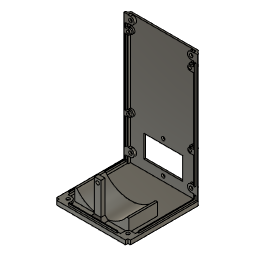
SolderingStation_Back (Autodesk Fusion 360 design; units mm, degrees)
Autodesk Fusion 360 part; units mm, degrees
sketch "Sketch1" plane through (0, 0, 0) normal (0, 0, 1) x (1, 0, 0)
  line L0 (45, 45) -> (-45, 45)
  line L1 (-45, 45) -> (-45, -45)
  line L2 (-45, -45) -> (45, -45)
  line L3 (45, -45) -> (45, 45)
  line L4 (45, 45) -> (-45, -45) construction
  line L5 (-45, 45) -> (45, -45) construction
  line L6 (-45, 45) -> (-42, 45) construction
  line L7 (-42, 45) -> (-42, 42)
  line L8 (-42, 42) -> (-45, 42)
  line L9 (0, 45) -> (0, -45) construction
  line L10 (-45, 0) -> (45, 0) construction
  line L11 (42, 45) -> (42, 42)
  line L12 (42, 42) -> (45, 42)
  line L13 (42, -42) -> (45, -42)
  line L14 (42, -45) -> (42, -42)
  line L15 (-42, -45) -> (-42, -42)
  line L16 (-42, -42) -> (-45, -42)
  dimension "d1" = 90
  dimension "d2" = 90
  constraint horizontal L0
  constraint perpendicular L0 L1
  constraint parallel L0 L2
  constraint parallel L1 L3
  constraint coincident L4 origin
  constraint coincident L5 origin
  constraint coincident L0 L6.end
  constraint coincident L5 L7.end
  constraint perpendicular L0 L7
  constraint coincident L1 L8.end
  constraint perpendicular L1 L8
  constraint midpoint L0 L9.start
  constraint midpoint L2 L9.end
  constraint midpoint L1 L10.start
  constraint midpoint L3 L10.end
  constraint symmetric L6.end L9 L11.start
  constraint symmetric L7.end L9 L11.end
  constraint symmetric L8.end L9 L12.end
  constraint symmetric L6.end L10 L15.start
  constraint symmetric L7.end L10 L15.end
  constraint symmetric L8.end L10 L16.end
  constraint symmetric L10 L11.start L14.start
  constraint symmetric L10 L11.end L13.start
  constraint symmetric L10 L12.end L13.end
  measures "d1" distance of L1.end L2.end
  measures "d2" distance of L0.end L1.end
extrude "Extrude1" add sketch "Sketch1" along normal blind 5 contours L0 L1 L2 L3 L7 L8 L11 L12 L13 L14 L15 L16 makes body 1
sketch "Sketch2" plane through (0, 0, 5) normal (0, 0, 1) x (-1, 0, 0)
  line L0 (42, 45) -> (-42, 45)
  line L1 (-42, 45) -> (-42, 42)
  line L2 (-42, 42) -> (-45, 42)
  line L3 (-45, 42) -> (-45, -42)
  line L4 (-45, -42) -> (-42, -42)
  line L5 (-42, -42) -> (-42, -45)
  line L6 (-42, -45) -> (42, -45)
  line L7 (42, -45) -> (42, -42)
  line L8 (42, -42) -> (45, -42)
  line L9 (45, -42) -> (45, 42)
  line L10 (45, 42) -> (42, 42)
  line L11 (42, 42) -> (42, 45)
  line L12 (38, -38) -> (41, -38)
  line L13 (41, -38) -> (41, 38)
  line L14 (41, 38) -> (38, 38)
  line L15 (38, 38) -> (38, 41)
  line L16 (38, 41) -> (-38, 41)
  line L17 (-38, 41) -> (-38, 38)
  line L18 (-38, 38) -> (-41, 38)
  line L19 (-41, 38) -> (-41, -38)
  line L20 (-41, -38) -> (-38, -38)
  line L21 (-38, -38) -> (-38, -41)
  line L22 (-38, -41) -> (38, -41)
  line L23 (38, -41) -> (38, -38)
  dimension "d5" = -4
extrude "Extrude2" cut sketch "Sketch2" against normal blind 3 contours L12 L13 L14 L15 L16 L17 L18 L19 L20 L21 L22 L23 bodies 1
sketch "Sketch3" plane through (0, 0, 5) normal (0, 0, 1) x (-1, 0, 0)
  line L0 (42, 45) -> (-42, 45)
  line L1 (-42, 45) -> (-42, 42)
  line L2 (-42, 42) -> (-45, 42)
  line L3 (-45, 42) -> (-45, -42)
  line L4 (-45, -42) -> (-42, -42)
  line L5 (-42, -42) -> (-42, -45)
  line L6 (-42, -45) -> (42, -45)
  line L7 (42, -45) -> (42, -42)
  line L8 (42, -42) -> (45, -42)
  line L9 (45, -42) -> (45, 42)
  line L10 (45, 42) -> (42, 42)
  line L11 (42, 42) -> (42, 45)
  line L12 (-39, 39) -> (-39, 42)
  line L13 (-39, 42) -> (39, 42)
  line L14 (39, 42) -> (39, 39)
  line L15 (39, 39) -> (42, 39)
  line L16 (42, 39) -> (42, -39)
  line L17 (42, -39) -> (39, -39)
  line L18 (39, -39) -> (39, -42)
  line L19 (39, -42) -> (-39, -42)
  line L20 (-39, -42) -> (-39, -39)
  line L21 (-39, -39) -> (-42, -39)
  line L22 (-42, -39) -> (-42, 39)
  line L23 (-42, 39) -> (-39, 39)
  line L24 (-40, 40) -> (-40, 43)
  line L25 (-40, 43) -> (40, 43)
  line L26 (40, 43) -> (40, 40)
  line L27 (40, 40) -> (43, 40)
  line L28 (43, 40) -> (43, -40)
  line L29 (43, -40) -> (40, -40)
  line L30 (40, -40) -> (40, -43)
  line L31 (40, -43) -> (-40, -43)
  line L32 (-40, -43) -> (-40, -40)
  line L33 (-40, -40) -> (-43, -40)
  line L34 (-43, -40) -> (-43, 40)
  line L35 (-43, 40) -> (-40, 40)
  line L36 (42, -39) -> (42, -40)
  line L37 (-42, -39) -> (-42, -40)
  line L38 (41, -38) -> (38, -38)
  line L39 (38, -38) -> (38, -41)
  line L40 (38, -41) -> (-38, -41)
  line L41 (-38, -41) -> (-38, -38)
  line L42 (-38, -38) -> (-41, -38)
  line L43 (-41, -38) -> (-41, 38)
  line L44 (-41, 38) -> (-38, 38)
  line L45 (-38, 38) -> (-38, 41)
  line L46 (-38, 41) -> (38, 41)
  line L47 (38, 41) -> (38, 38)
  line L48 (38, 38) -> (41, 38)
  line L49 (41, 38) -> (41, -38)
  constraint coincident L29 L36.end
  constraint perpendicular L29 L36
  constraint coincident L33 L37.end
  constraint perpendicular L33 L37
extrude "Extrude3" add sketch "Sketch3" along normal blind 2 contours L12 L13 L14 L15 L16 L22 L23 L24 L25 L26 L27 L28 L29 L33 L34 L35 L36 L37 bodies 1
fillet "Fillet1" radius 1 7 edges at (-42, 0.5, 5) (42, 0.5, 5) (40.5, -39, 5) (39, -40.5, 5) (0, -42, 5) (-39, -40.5, 5) (-40.5, -39, 5) on bodies 1
sketch "Sketch4" plane through (0, 0, 0) normal (0, 0, -1) x (1, 0, 0)
  line L0 (42, 45) -> (-42, 45)
  line L1 (-42, 45) -> (-42, 42)
  line L2 (-42, 42) -> (-45, 42)
  line L3 (-45, 42) -> (-45, -42)
  line L4 (-45, -42) -> (-42, -42)
  line L5 (-42, -42) -> (-42, -45)
  line L6 (-42, -45) -> (42, -45)
  line L7 (42, -45) -> (42, -42)
  line L8 (42, -42) -> (45, -42)
  line L9 (45, -42) -> (45, 42)
  line L10 (45, 42) -> (42, 42)
  line L11 (42, 42) -> (42, 45)
  line L12 (-45, -40) -> (-40, -40)
  line L13 (-40, -40) -> (-40, -43)
  line L14 (-40, -43) -> (40, -43)
  line L15 (40, -43) -> (40, -40)
  line L16 (40, -40) -> (45, -40)
  dimension "d14" = -2
extrude "Extrude4" add sketch "Sketch4" against normal blind 160 contours L3 L4 L5 L6 L7 L8 L9 L12 L13 L14 L15 L16 bodies 1
extrude "Extrude5" cut 1 faces at (-12.6667, 42.3333, 5) along direction (0, 0, -1) blind 3 on bodies 1 bodies 1
sketch "Sketch5" plane through (0, 0, 2) normal (0, 0, 1) x (-1, 0, 0)
  line L0 (41, -40) -> (41, 38)
  line L1 (41, 38) -> (38, 38)
  line L2 (38, 38) -> (38, 41)
  line L3 (38, 41) -> (-38, 41)
  line L4 (-38, 41) -> (-38, 38)
  line L5 (-38, 38) -> (-41, 38)
  line L6 (-41, 38) -> (-41, -40)
  line L7 (-41, -40) -> (-40, -40)
  line L8 (-40, -40) -> (-40, -43)
  line L9 (-40, -43) -> (40, -43)
  line L10 (40, -43) -> (40, -40)
  line L11 (40, -40) -> (41, -40)
  line L12 (-44.9376, -44.9376) -> (44.9376, -44.9376) construction
  line L13 (44.9376, -44.9376) -> (44.9376, 44.9376) construction
  line L14 (44.9376, 44.9376) -> (-44.9376, 44.9376) construction
  line L15 (-44.9376, 44.9376) -> (-44.9376, -44.9376) construction
  line L16 (-44.9376, -44.9376) -> (44.9376, 44.9376) construction
  line L17 (44.9376, -44.9376) -> (-44.9376, 44.9376) construction
  circle A0 centre (36.4523, 36.4523) radius 2.15 construction
  circle A1 centre (36.4523, 36.4523) radius 2.15 construction
  circle A2 centre (36.4523, 36.4523) radius 2
  line L18 (0, 0) -> (0, 44.9376) construction
  circle A3 centre (-36.4523, 36.4523) radius 2.15 construction
  circle A4 centre (-36.4523, 36.4523) radius 2
  dimension "d19" = 4.3
  dimension "d20" = 12
  dimension "d27" = 4.3
  constraint horizontal L12
  constraint perpendicular L12 L13
  constraint parallel L12 L14
  constraint parallel L13 L15
  constraint coincident L16 L18.start
  constraint coincident L17 L18.start
  constraint coincident L18.start origin
  constraint coincident L16 A0.centre
  constraint concentric A0 A1
  constraint concentric A0 A2
  constraint midpoint L14 L18.end
  constraint symmetric A1 L18 A3
  constraint concentric A3 A4
  measures "d19" diameter of A0
  measures "d20" distance of L13.end A0.centre
  measures "d27" diameter of A3
extrude "Extrude6" cut sketch "Sketch5" against normal blind 3 contours A2 | A4 bodies 1
sketch "Sketch7" plane through (0, 0, 0) normal (0, 0, -1) x (1, 0, 0)
  circle A0 centre (-36.4523, 36.4523) radius 2
  circle A1 centre (36.4523, 36.4523) radius 2
  line L0 (45, -42) -> (45, 42)
  line L1 (45, 42) -> (42, 42)
  line L2 (42, 42) -> (42, 45)
  line L3 (42, 45) -> (-42, 45)
  line L4 (-42, 45) -> (-42, 42)
  line L5 (-42, 42) -> (-45, 42)
  line L6 (-45, 42) -> (-45, -42)
  line L7 (-45, -42) -> (-42, -42)
  line L8 (-42, -42) -> (-42, -45)
  line L9 (-42, -45) -> (42, -45)
  line L10 (42, -45) -> (42, -42)
  line L11 (42, -42) -> (45, -42)
  circle A2 centre (-36.4523, 36.4523) radius 4.5
  line L12 (-36.4523, 36.4523) -> (-31.9523, 36.4523) construction
  line L13 (-36.4523, 36.4523) -> (-36.4523, 31.9523) construction
  line L14 (-31.9523, 36.4523) -> (-31.9523, 45)
  line L15 (-36.4523, 31.9523) -> (-45, 31.9523)
  line L16 (43, -42) -> (43, 40)
  line L17 (43, 40) -> (40, 40)
  line L18 (40, 40) -> (40, 43)
  line L19 (40, 43) -> (-40, 43)
  line L20 (-40, 43) -> (-40, 40)
  line L21 (-40, 40) -> (-43, 40)
  line L22 (-43, 40) -> (-43, -42)
  line L23 (0, 45) -> (0, 26) construction
  circle A3 centre (36.4523, 36.4523) radius 4.5
  line L24 (31.9523, 36.4523) -> (31.9523, 45)
  line L25 (36.4523, 31.9523) -> (45, 31.9523)
  dimension "d23" = 9
  dimension "d24" = -2
  constraint concentric A0 A2
  constraint coincident A0.centre A2.centre
  constraint coincident A2 L12.end
  constraint horizontal L12
  constraint coincident A2 L13.end
  constraint perpendicular L12 L13
  constraint coincident L3 L14.end
  constraint tangent A2 L14
  constraint coincident L6 L15.end
  constraint tangent A2 L15
  constraint midpoint L3 L23.start
  constraint perpendicular L3 L23
  constraint symmetric A2 L23 A3
  constraint symmetric L12.end L23 L24.start
  constraint symmetric L13.end L23 L25.start
  constraint symmetric L14.end L23 L24.end
  constraint symmetric L15.end L23 L25.end
  measures "d23" diameter of A2
extrude "Extrude7" add sketch "Sketch7" against normal blind 7 contours L16 L17 L18 L19 A3 L24 L25 | A3 | A2 L14 L15 L19 L20 L21 L22 | A2 bodies 1
sketch "Sketch9" plane through (0, 45, 0) normal (0, 1, 0) x (-1, 0, 0)
  line L0 (-42, 0) -> (42, 0)
  line L1 (42, 0) -> (42, 160)
  line L2 (42, 160) -> (-42, 160)
  line L3 (-42, 160) -> (-42, 0)
  line L4 (0, 0) -> (0, 67.5) construction
  line L5 (23.65, 41.15) -> (-23.65, 41.15)
  line L6 (-23.65, 41.15) -> (-23.65, 13.85)
  line L7 (-23.65, 13.85) -> (23.65, 13.85)
  line L8 (23.65, 13.85) -> (23.65, 41.15)
  line L9 (23.65, 41.15) -> (-23.65, 13.85) construction
  line L10 (-23.65, 41.15) -> (23.65, 13.85) construction
  circle A0 centre (0, 47.2) radius 2.15
  line L11 (0, 27.5) -> (-23.65, 27.5) construction
  circle A1 centre (0, 7.8) radius 2.15
  point P0 (0, 27.5)
  dimension "d28" = 47.3
  dimension "d29" = 27.3
  dimension "d30" = 27.5
  dimension "d31" = 4.3
  dimension "d33" = 19.7
  constraint coincident L4.start origin
  constraint perpendicular L0 L4
  constraint horizontal L5
  constraint perpendicular L5 L6
  constraint parallel L5 L7
  constraint parallel L6 L8
  constraint coincident L9 P0
  constraint coincident L10 P0
  constraint coincident L4 P0
  constraint coincident L4 A0.centre
  constraint coincident P0 L11.start
  constraint midpoint L6 L11.end
  constraint symmetric A0 L11 A1
  measures "d28" distance of L6.end L7.end
  measures "d29" distance of L5.end L6.end
  measures "d30" distance of L0 P0
  measures "d31" diameter of A0
  measures "d33" distance of A0.centre L11
extrude "Extrude8" cut sketch "Sketch9" against normal blind 2 contours L5 L6 L7 L8 | A0 | A1 bodies 1
sketch "Sketch10" plane through (0, 45, 0) normal (0, 1, 0) x (-1, 0, 0)
  circle A0 centre (0, 7.8) radius 2.15
  line L0 (-23.65, 41.15) -> (23.65, 41.15)
  line L1 (23.65, 41.15) -> (23.65, 13.85)
  line L2 (23.65, 13.85) -> (-23.65, 13.85)
  line L3 (-23.65, 13.85) -> (-23.65, 41.15)
  circle A1 centre (0, 47.2) radius 2.15
  line L4 (-42, 0) -> (42, 0)
  line L5 (42, 0) -> (42, 160)
  line L6 (42, 160) -> (-42, 160)
  line L7 (-42, 160) -> (-42, 0)
  circle A2 centre (-37, 15) radius 4.5
  line L8 (-45, 0) -> (-45, 160)
  circle A3 centre (-37, 15) radius 2.15
  line L9 (-37, 15) -> (-37, 19.5) construction
  line L10 (-37, 15) -> (-37, 10.5) construction
  line L11 (-37, 19.5) -> (-42, 19.5)
  line L12 (-37, 10.5) -> (-42, 10.5)
  line L13 (0, 0) -> (0, 47.2) construction
  circle A4 centre (37, 15) radius 4.5
  circle A5 centre (37, 15) radius 2.15
  line L14 (37, 10.5) -> (42, 10.5)
  line L15 (37, 19.5) -> (42, 19.5)
  circle A6 centre (37, 15) radius 2.15
  circle A7 centre (37, 15) radius 4.5
  line L16 (37, 19.5) -> (42, 19.5)
  line L17 (37, 10.5) -> (42, 10.5)
  line L18 (-37, 19.5) -> (-42, 19.5)
  circle A8 centre (-37, 15) radius 4.5
  circle A9 centre (-37, 15) radius 2.15
  circle A10 centre (-37, 155) radius 4.5
  line L19 (-37, 150.5) -> (-42, 150.5)
  circle A11 centre (-37, 155) radius 2.15
  line L20 (-37, 159.5) -> (-42, 159.5)
  line L21 (37, 150.5) -> (42, 150.5)
  circle A12 centre (37, 155) radius 4.5
  line L22 (37, 159.5) -> (42, 159.5)
  circle A13 centre (37, 155) radius 2.15
  dimension "d36" = 9
  dimension "d37" = 15
  dimension "d38" = 8
  dimension "d39" = 4.3
  dimension "d40" = 9
  dimension "d41" = 4.3
  dimension "d42" = 9
  dimension "d43" = 4.3
  constraint concentric A2 A3
  constraint coincident A2.centre A3.centre
  constraint coincident A2 L9.end
  constraint vertical L9
  constraint coincident A2 L10.end
  constraint parallel L9 L10
  constraint coincident L7 L11.end
  constraint tangent A2 L11
  constraint coincident L7 L12.end
  constraint tangent A2 L12
  constraint coincident L13.start origin
  constraint coincident A1.centre L13.end
  constraint symmetric A2 L13 A4
  constraint symmetric A3 L13 A5
  constraint symmetric L9.end L13 L15.start
  constraint symmetric L10.end L13 L14.start
  constraint symmetric L11.end L13 L15.end
  constraint symmetric L12.end L13 L14.end
  constraint concentric A8 A9
  constraint coincident L9.end A8
  constraint tangent L18 A8
  constraint concentric A10 A11
  constraint coincident L20.start A10
  constraint tangent A10 L20
  measures "d36" diameter of A2
  measures "d37" distance of L4 A2.centre
  measures "d38" distance of A2.centre L8
  measures "d39" diameter of A3
  measures "d40" diameter of A8
  measures "d41" diameter of A9
  measures "d42" diameter of A10
  measures "d43" diameter of A11
extrude "Extrude9" add sketch "Sketch10" against normal blind 7 contours L7 A2 L11 L12 L18 A8 | L5 A4 L14 L15 A7 L16 L17 | A2 A8 | A4 A7 | L7 A10 L19 L20 | L5 L21 A12 L22 | A10 | A12 bodies 1
sketch "Sketch11" plane through (0, 40, 0) normal (0, -1, 0) x (1, 0, 0)
  line L0 (40, 19.5) -> (42, 19.5)
  line L1 (42, 19.5) -> (42, 10.5)
  line L2 (42, 10.5) -> (40, 10.5)
  line L3 (40, 10.5) -> (40, 2)
  line L4 (40, 2) -> (41, 2)
  line L5 (41, 2) -> (41, 5)
  arc A0 (41, 5) -> (42, 6) centre (41, 6) ccw
  line L6 (42, 6) -> (42, 7)
  line L7 (42, 7) -> (43, 7)
  line L8 (43, 7) -> (43, 5)
  line L9 (43, 5) -> (45, 5)
  line L10 (45, 5) -> (45, 160)
  line L11 (45, 160) -> (40, 160)
  line L12 (40, 160) -> (40, 159.5)
  line L13 (40, 159.5) -> (42, 159.5)
  line L14 (42, 159.5) -> (42, 150.5)
  line L15 (42, 150.5) -> (40, 150.5)
  line L16 (40, 150.5) -> (40, 19.5)
  line L17 (43, 5) -> (43, 160)
  line L18 (42, 5) -> (42, 160)
  line L19 (0, 41) -> (0, 14) construction
  line L20 (-42, 5) -> (-42, 160)
  line L21 (-43, 5) -> (-43, 160)
  line L22 (-42, 5) -> (-43, 5)
  line L23 (-43, 160) -> (-42, 160)
  constraint coincident L8.end L9.start
  constraint coincident L11 L17.end
  constraint perpendicular L11 L17
  constraint coincident L11 L18.end
  constraint perpendicular L11 L18
  constraint vertical L19
  constraint vertical L20
  constraint parallel L20 L21
  constraint perpendicular L21 L22
  constraint perpendicular L20 L23
extrude "Extrude10" add sketch "Sketch11" along normal blind 2 contours L1 L7 L11 L14 L17 L18 | L20 L21 L22 L23 bodies 1
fillet "Fillet2" radius 1 6 edges at (-41.7071, 40, 5.2929) (-42, 40, 8.25) (-42, 40, 85) (42, 40, 85) (41.7071, 40, 5.2929) (42, 40, 8.25) on bodies 1
extrude "Extrude11" cut 4 faces at (37.6599, 43, 15.5763) (-36.4428, 43, 14.7238) (-36.6417, 43, 155.6207) (36.4461, 43, 155.5603) along direction (0, 1, 0) blind 2 on bodies 1 bodies 1
sketch "Sketch12" plane through (0, 0, 0) normal (0, 0, -1) x (1, 0, 0)
  circle A0 centre (-36.4523, 36.4523) radius 2
  circle A1 centre (36.4523, 36.4523) radius 2
  line L0 (45, -42) -> (45, 42)
  line L1 (45, 42) -> (42, 42)
  line L2 (42, 42) -> (42, 45)
  line L3 (42, 45) -> (-42, 45)
  line L4 (-42, 45) -> (-42, 42)
  line L5 (-42, 42) -> (-45, 42)
  line L6 (-45, 42) -> (-45, -42)
  line L7 (-45, -42) -> (-42, -42)
  line L8 (-42, -42) -> (-42, -45)
  line L9 (-42, -45) -> (42, -45)
  line L10 (42, -45) -> (42, -42)
  line L11 (42, -42) -> (45, -42)
  circle A2 centre (-36.4523, 36.4523) radius 3.75
  circle A3 centre (36.4523, 36.4523) radius 3.75
  dimension "d52" = 7.5
  dimension "d53" = 7.5
  constraint concentric A0 A2
  constraint concentric A1 A3
  measures "d52" diameter of A2
  measures "d53" diameter of A3
extrude "Extrude12" cut sketch "Sketch12" against normal blind 3 contours A2 | A3 bodies 1
sketch "Sketch13" plane through (0, 45, 0) normal (0, 1, 0) x (-1, 0, 0)
  circle A0 centre (37, 155) radius 2.15
  circle A1 centre (-37, 15) radius 2.15
  circle A2 centre (37, 15) radius 2.15
  circle A3 centre (-37, 155) radius 2.15
  circle A4 centre (0, 47.2) radius 2.15
  line L0 (-23.65, 41.15) -> (23.65, 41.15)
  line L1 (23.65, 41.15) -> (23.65, 13.85)
  line L2 (23.65, 13.85) -> (-23.65, 13.85)
  line L3 (-23.65, 13.85) -> (-23.65, 41.15)
  circle A5 centre (0, 7.8) radius 2.15
  line L4 (-42, 160) -> (-42, 0)
  line L5 (-42, 0) -> (42, 0)
  line L6 (42, 0) -> (42, 160)
  line L7 (42, 160) -> (-42, 160)
  circle A6 centre (-37, 155) radius 3.75
  circle A7 centre (37, 155) radius 3.75
  circle A8 centre (37, 15) radius 3.75
  circle A9 centre (-37, 15) radius 3.75
  dimension "d56" = 7.5
  dimension "d57" = 7.5
  dimension "d58" = 7.5
  dimension "d59" = 7.5
  constraint concentric A3 A6
  constraint concentric A0 A7
  constraint concentric A2 A8
  constraint concentric A1 A9
  measures "d56" diameter of A6
  measures "d57" diameter of A7
  measures "d58" diameter of A8
  measures "d59" diameter of A9
extrude "Extrude13" cut sketch "Sketch13" against normal blind 3 contours A6 | A7 | A8 | A9 bodies 1
sketch "Sketch14" plane through (0, 43, 0) normal (0, -1, 0) x (1, 0, 0)
  line L0 (37, 19.5) -> (40, 19.5)
  line L1 (40, 19.5) -> (40, 150.5)
  line L2 (40, 150.5) -> (37, 150.5)
  arc A0 (37, 159.5) -> (37, 150.5) centre (37, 155) ccw
  line L3 (37, 159.5) -> (40, 159.5)
  line L4 (40, 159.5) -> (40, 160)
  line L5 (40, 160) -> (-40, 160)
  line L6 (-40, 160) -> (-40, 159.5)
  line L7 (-40, 159.5) -> (-37, 159.5)
  arc A1 (-37, 150.5) -> (-37, 159.5) centre (-37, 155) ccw
  line L8 (-37, 150.5) -> (-40, 150.5)
  line L9 (-40, 150.5) -> (-40, 19.5)
  line L10 (-40, 19.5) -> (-37, 19.5)
  arc A2 (-37, 10.5) -> (-37, 19.5) centre (-37, 15) ccw
  line L11 (-37, 10.5) -> (-40, 10.5)
  line L12 (-40, 10.5) -> (-40, 2)
  line L13 (-40, 2) -> (40, 2)
  line L14 (40, 2) -> (40, 10.5)
  line L15 (40, 10.5) -> (37, 10.5)
  arc A3 (37, 19.5) -> (37, 10.5) centre (37, 15) ccw
  circle A4 centre (0, 47.2) radius 2.15
  line L16 (-23.65, 41.15) -> (23.65, 41.15)
  line L17 (23.65, 41.15) -> (23.65, 13.85)
  line L18 (23.65, 13.85) -> (-23.65, 13.85)
  line L19 (-23.65, 13.85) -> (-23.65, 41.15)
  circle A5 centre (0, 7.8) radius 2.15
  line L20 (0, 160) -> (0, 0) construction
  line L21 (40.965, 146.53) -> (-40.965, 146.53) construction
  line L22 (-40.965, 146.53) -> (-40.965, 53.47) construction
  line L23 (-40.965, 53.47) -> (40.965, 53.47) construction
  line L24 (40.965, 53.47) -> (40.965, 146.53) construction
  line L25 (40.965, 146.53) -> (-40.965, 53.47) construction
  line L26 (-40.965, 146.53) -> (40.965, 53.47) construction
  point P0 (0, 100)
  dimension "d62" = 81.93
  dimension "d63" = 93.06
  dimension "d64" = 60
  constraint midpoint L5 L20.start
  constraint coincident L20.end origin
  constraint horizontal L21
  constraint perpendicular L21 L22
  constraint parallel L21 L23
  constraint parallel L22 L24
  constraint coincident L25 P0
  constraint coincident L26 P0
  constraint coincident L20 P0
  measures "d62" distance of L22.end L23.end
  measures "d63" distance of L21.end L22.end
  measures "d64" distance of L5 P0
sketch "Sketch15" plane through (0, 45, 0) normal (0, 1, 0) x (-1, 0, 0)
  circle A0 centre (37, 15) radius 3.75
  circle A1 centre (37, 155) radius 3.75
  circle A2 centre (-37, 15) radius 3.75
  circle A3 centre (-37, 155) radius 3.75
  circle A4 centre (0, 47.2) radius 2.15
  line L0 (-23.65, 41.15) -> (23.65, 41.15)
  line L1 (23.65, 41.15) -> (23.65, 13.85)
  line L2 (23.65, 13.85) -> (-23.65, 13.85)
  line L3 (-23.65, 13.85) -> (-23.65, 41.15)
  circle A5 centre (0, 7.8) radius 2.15
  line L4 (-42, 160) -> (-42, 0)
  line L5 (-42, 0) -> (42, 0)
  line L6 (42, 0) -> (42, 160)
  line L7 (42, 160) -> (-42, 160)
  line L8 (40.965, 146.53) -> (-40.965, 146.53)
  line L9 (-40.965, 146.53) -> (-40.965, 53.47)
  line L10 (-40.965, 53.47) -> (40.965, 53.47)
  line L11 (40.965, 53.47) -> (40.965, 146.53)
  line L12 (40.965, 146.53) -> (-40.965, 53.47) construction
  line L13 (-40.965, 146.53) -> (40.965, 53.47) construction
  circle A6 centre (-37.765, 143.33) radius 1.65
  circle A7 centre (38.265, 143.23) radius 1.65
  circle A8 centre (-37.915, 56.17) radius 1.65
  circle A9 centre (38.165, 56.17) radius 1.65
  circle A10 centre (-37.765, 143.33) radius 3
  circle A11 centre (38.265, 143.23) radius 3
  circle A12 centre (38.165, 56.17) radius 3
  circle A13 centre (-37.915, 56.17) radius 3
  line L14 (-37.915, 56.17) -> (-37.915, 59.17) construction
  line L15 (-37.915, 56.17) -> (-37.915, 53.17) construction
  line L16 (-37.915, 59.17) -> (-42, 59.17)
  line L17 (-37.915, 53.17) -> (-42, 53.17)
  line L18 (38.165, 56.17) -> (38.165, 59.17) construction
  line L19 (38.165, 56.17) -> (38.165, 53.17) construction
  line L20 (38.165, 53.17) -> (42, 53.17)
  line L21 (38.165, 59.17) -> (42, 59.17)
  line L22 (38.265, 143.23) -> (38.265, 146.23) construction
  line L23 (38.265, 143.23) -> (38.265, 140.23) construction
  line L24 (38.265, 140.23) -> (42, 140.23)
  line L25 (38.265, 146.23) -> (42, 146.23)
  line L26 (-37.765, 143.33) -> (-37.765, 146.33) construction
  line L27 (-37.765, 143.33) -> (-37.765, 140.33) construction
  line L28 (-37.765, 140.33) -> (-42, 140.33)
  line L29 (-37.765, 146.33) -> (-42, 146.33)
  point P0 (0, 100)
  dimension "d65" = 81.93
  dimension "d66" = 93.06
  dimension "d67" = 60
  dimension "d70" = 3.3
  dimension "d71" = 3.2
  dimension "d72" = 3.2
  dimension "d73" = 3.3
  dimension "d74" = 2.7
  dimension "d75" = 3.3
  dimension "d76" = 3.3
  dimension "d77" = 2.7
  dimension "d78" = 3.05
  dimension "d79" = 3.3
  dimension "d80" = 2.8
  dimension "d81" = 2.7
  dimension "d82" = 6
  dimension "d83" = 6
  dimension "d84" = 6
  dimension "d85" = 6
  constraint horizontal L8
  constraint perpendicular L8 L9
  constraint parallel L8 L10
  constraint parallel L9 L11
  constraint coincident L12 P0
  constraint coincident L13 P0
  constraint concentric A6 A10
  constraint concentric A7 A11
  constraint concentric A9 A12
  constraint concentric A8 A13
  constraint coincident A8.centre A13.centre
  constraint coincident A13 L14.end
  constraint vertical L14
  constraint coincident A13 L15.end
  constraint perpendicular L10 L15
  constraint coincident L4 L16.end
  constraint tangent A13 L16
  constraint coincident L4 L17.end
  constraint tangent A13 L17
  constraint coincident A9.centre A12.centre
  constraint coincident A12 L18.end
  constraint perpendicular L17 L18
  constraint coincident A12 L19.end
  constraint perpendicular L10 L19
  constraint coincident L6 L20.end
  constraint tangent A12 L20
  constraint coincident L6 L21.end
  constraint tangent A12 L21
  constraint coincident A7.centre A11.centre
  constraint coincident A11 L22.end
  constraint perpendicular L21 L22
  constraint coincident A11 L23.end
  constraint parallel L22 L23
  constraint coincident L6 L24.end
  constraint tangent A11 L24
  constraint coincident L6 L25.end
  constraint tangent A11 L25
  constraint coincident A6.centre A10.centre
  constraint coincident A10 L26.end
  constraint perpendicular L25 L26
  constraint coincident A10 L27.end
  constraint parallel L26 L27
  constraint coincident L4 L28.end
  constraint tangent A10 L28
  constraint coincident L4 L29.end
  constraint tangent A10 L29
  measures "d65" distance of L9.end L10.end
  measures "d66" distance of L8.end L9.end
  measures "d67" distance of L7 P0
  measures "d70" diameter of A6
  measures "d71" distance of L8 A6.centre
  measures "d72" distance of L9 A6.centre
  measures "d73" diameter of A7
  measures "d74" distance of L11 A7.centre
  measures "d75" distance of L8 A7.centre
  measures "d76" diameter of A8
  measures "d77" distance of L10 A8.centre
  measures "d78" distance of L9 A8.centre
  measures "d79" diameter of A9
  measures "d80" distance of L11 A9.centre
  measures "d81" distance of L10 A9.centre
  measures "d82" diameter of A10
  measures "d83" diameter of A11
  measures "d84" diameter of A12
  measures "d85" diameter of A13
extrude "Extrude14" add sketch "Sketch15" against normal blind 7 contours L4 L9 L28 L29 | L9 A10 L28 L29 | L6 L11 A11 L24 L25 | L4 L9 L10 A13 L16 L17 | A10 | L11 A11 L25 | L9 L10 A13 L16 | L6 L10 L11 A12 L20 L21 | L11 A11 L24 | L11 A11 | L11 A11 | L10 A13 | L10 A13 | L11 A12 L21 | L10 A12 | L11 A12 | L10 L11 A12 | L10 L11 A12 bodies 1
extrude "Extrude15" cut 4 faces at (-38.0426, 43, 56.7062) (37.6319, 43, 56.682) (37.1773, 43, 143.76) (-38.1426, 43, 143.7662) along direction (0, 1, 0) blind 2 on bodies 1 bodies 1
sketch "Sketch18" plane through (0, 45, 0) normal (0, 1, 0) x (-1, 0, 0)
  circle A0 centre (-37.765, 143.33) radius 1.65
  circle A1 centre (38.165, 56.17) radius 1.65
  circle A2 centre (-37.915, 56.17) radius 1.65
  circle A3 centre (38.265, 143.23) radius 1.65
  circle A4 centre (0, 7.8) radius 2.15
  line L0 (-23.65, 41.15) -> (23.65, 41.15)
  line L1 (23.65, 41.15) -> (23.65, 13.85)
  line L2 (23.65, 13.85) -> (-23.65, 13.85)
  line L3 (-23.65, 13.85) -> (-23.65, 41.15)
  circle A5 centre (0, 47.2) radius 2.15
  circle A6 centre (-37, 155) radius 3.75
  circle A7 centre (-37, 15) radius 3.75
  circle A8 centre (37, 155) radius 3.75
  circle A9 centre (37, 15) radius 3.75
  line L4 (-42, 160) -> (-42, 0)
  line L5 (-42, 0) -> (42, 0)
  line L6 (42, 0) -> (42, 160)
  line L7 (42, 160) -> (-42, 160)
  circle A10 centre (38.165, 56.17) radius 3.835
  circle A11 centre (-37.915, 56.17) radius 4.085
  circle A12 centre (-37.765, 143.33) radius 4.235
  circle A13 centre (38.265, 143.23) radius 3.735
  constraint concentric A1 A10
  constraint tangent L6 A10
  constraint concentric A2 A11
  constraint tangent L4 A11
  constraint concentric A0 A12
  constraint tangent L4 A12
  constraint concentric A3 A13
  constraint tangent L6 A13
extrude "Extrude16" add sketch "Sketch18" against normal blind 4 contours A12 | A11 | A10 | A13 bodies 1
fillet "Fillet3" radius 1 12 edges at (38.9575, 41, 59.17) (34.915, 41, 56.17) (38.9575, 41, 53.17) (38.8825, 41, 146.33) (34.765, 41, 143.33) (38.8825, 41, 140.33) (-39.1325, 41, 140.23) (-35.265, 41, 143.23) (-39.1325, 41, 146.23) (-39.0825, 41, 53.17) (-35.165, 41, 56.17) (-39.0825, 41, 59.17) on bodies 1
sketch "Sketch17" plane through (0, 45, 0) normal (0, 1, 0) x (-1, 0, 0)
  circle A0 centre (-37.765, 143.33) radius 1.65
  circle A1 centre (38.165, 56.17) radius 1.65
  circle A2 centre (-37.915, 56.17) radius 1.65
  circle A3 centre (38.265, 143.23) radius 1.65
  circle A4 centre (0, 7.8) radius 2.15
  line L0 (-23.65, 41.15) -> (23.65, 41.15)
  line L1 (23.65, 41.15) -> (23.65, 13.85)
  line L2 (23.65, 13.85) -> (-23.65, 13.85)
  line L3 (-23.65, 13.85) -> (-23.65, 41.15)
  circle A5 centre (0, 47.2) radius 2.15
  circle A6 centre (-37, 155) radius 3.75
  circle A7 centre (-37, 15) radius 3.75
  circle A8 centre (37, 155) radius 3.75
  circle A9 centre (37, 15) radius 3.75
  line L4 (-42, 160) -> (-42, 0)
  line L5 (-42, 0) -> (42, 0)
  line L6 (42, 0) -> (42, 160)
  line L7 (42, 160) -> (-42, 160)
  circle A10 centre (-37.765, 143.33) radius 3.1
  circle A11 centre (38.265, 143.23) radius 3.1
  circle A12 centre (38.165, 56.17) radius 3.1
  circle A13 centre (-37.915, 56.17) radius 3.1
  dimension "d90" = 6.2
  dimension "d91" = 6.2
  dimension "d92" = 6.2
  dimension "d93" = 6.2
  constraint concentric A0 A10
  constraint concentric A3 A11
  constraint concentric A1 A12
  constraint concentric A2 A13
  measures "d90" diameter of A10
  measures "d91" diameter of A11
  measures "d92" diameter of A12
  measures "d93" diameter of A13
extrude "Extrude17" cut sketch "Sketch17" against normal blind 2 contours A10 | A11 | A12 | A13 bodies 1
sketch "Sketch20" plane through (0, 0, 0) normal (0, 0, -1) x (1, 0, 0)
  circle A0 centre (-36.4523, 36.4523) radius 3.75
  circle A1 centre (36.4523, 36.4523) radius 3.75
  line L0 (45, -42) -> (45, 42)
  line L1 (45, 42) -> (42, 42)
  line L2 (42, 42) -> (42, 45)
  line L3 (42, 45) -> (-42, 45)
  line L4 (-42, 45) -> (-42, 42)
  line L5 (-42, 42) -> (-45, 42)
  line L6 (-45, 42) -> (-45, -42)
  line L7 (-45, -42) -> (-42, -42)
  line L8 (-42, -42) -> (-42, -45)
  line L9 (-42, -45) -> (42, -45)
  line L10 (42, -45) -> (42, -42)
  line L11 (42, -42) -> (45, -42)
  line L12 (0, 45) -> (0, -45) construction
  line L13 (42, -42) -> (42, 42) construction
  line L14 (-42, 42) -> (-42, -42) construction
  line L15 (-33, 32) -> (33, 32)
  line L16 (33, 32) -> (33, -3)
  line L17 (33, -3) -> (-33, -3)
  line L18 (-33, -3) -> (-33, 32)
  line L19 (-33, 32) -> (33, -3) construction
  line L20 (33, 32) -> (-33, -3) construction
  point P0 (0, 14.5)
  dimension "d101" = 35
  dimension "d102" = 13
  dimension "d114" = 66
  constraint midpoint L3 L12.start
  constraint midpoint L9 L12.end
  constraint coincident L10.end L11.start
  constraint coincident L1.end L2.start
  constraint coincident L4.end L5.start
  constraint coincident L7.end L8.start
  constraint horizontal L15
  constraint perpendicular L15 L16
  constraint parallel L15 L17
  constraint parallel L16 L18
  constraint coincident L19 P0
  constraint coincident L20 P0
  constraint coincident L12 P0
  measures "d101" distance of L15.end L16.end
  measures "d102" distance of L3 L15
  measures "d114" distance of L16.end L17.end
extrude "Extrude18" add sketch "Sketch20" against normal blind 7 contours L15 L16 L17 L18 bodies 1
sketch "Sketch21" plane through (0, 0, 7) normal (0, 0, 1) x (-1, 0, 0)
  arc A0 (-36.4523, 31.9523) -> (-31.9523, 36.4523) centre (-36.4523, 36.4523) ccw
  line L0 (-31.9523, 36.4523) -> (-31.9523, 42)
  line L1 (-31.9523, 42) -> (31.9523, 42)
  line L2 (31.9523, 42) -> (31.9523, 36.4523)
  arc A1 (31.9523, 36.4523) -> (36.4523, 31.9523) centre (36.4523, 36.4523) ccw
  line L3 (42, 31.9523) -> (42, -38)
  line L4 (42, -38) -> (43, -38)
  line L5 (43, -38) -> (43, 40)
  line L6 (43, 40) -> (40, 40)
  line L7 (40, 40) -> (40, 43)
  line L8 (40, 43) -> (-40, 43)
  line L9 (-40, 43) -> (-40, 40)
  line L10 (-40, 40) -> (-43, 40)
  line L11 (-43, 40) -> (-43, -38)
  line L12 (-43, -38) -> (-42, -38)
  line L13 (-42, -38) -> (-42, 31.9523)
  circle A2 centre (36.4523, 36.4523) radius 2
  circle A3 centre (-36.4523, 36.4523) radius 2
  line L14 (0, -3) -> (0, 32) construction
  line L15 (0, 14.5) -> (43, 14.5) construction
  line L16 (43, -3) -> (-43, -3)
  line L17 (-43, -3) -> (-43, 32)
  line L18 (-43, 32) -> (43, 32)
  line L19 (43, 32) -> (43, -3)
  line L20 (43, -3) -> (-43, 32) construction
  line L21 (-43, -3) -> (43, 32) construction
  line L22 (-42, 31.9523) -> (-36.4523, 31.9523)
  line L23 (36.4523, 31.9523) -> (42, 31.9523)
  point P0 (0, 14.5)
  constraint midpoint L14 P0
  constraint coincident L5 L15.end
  constraint perpendicular L5 L15
  constraint horizontal L16
  constraint perpendicular L16 L17
  constraint parallel L16 L18
  constraint parallel L17 L19
  constraint coincident L5 L16.start
  constraint coincident L20 P0
  constraint coincident L21 P0
  constraint coincident P0 L15.start
extrude "Extrude19" add sketch "Sketch21" along normal blind 10 contours A0 L11 L13 L16 L17 L18 L22 | A0 A1 L3 L13 L16 L18 L22 L23 | A1 L3 L5 L16 L18 L19 L23 bodies 1
sketch "Sketch22" plane through (0, -32, 0) normal (0, -1, 0) x (1, 0, 0)
  line L0 (35.7991, 7) -> (43, 7)
  line L1 (43, 7) -> (43, 17)
  line L2 (43, 17) -> (-43, 17)
  line L3 (-43, 17) -> (-43, 7)
  line L4 (-33, 2) -> (33, 2)
  line L5 (0, 2) -> (0, 72) construction
  circle A0 centre (0, 40.5) radius 38.5
  line L6 (0, 2) -> (-13, 2) construction
  line L7 (33, 2) -> (33, 7)
  line L8 (33, 7) -> (35.7991, 7)
  line L9 (-43, 7) -> (-35.7991, 7)
  line L10 (-35.7991, 7) -> (-33, 7)
  line L11 (-33, 7) -> (-33, 2)
  dimension "d107" = 77
  constraint midpoint L4 L5.start
  constraint perpendicular L4 L5
  constraint coincident L5 A0.centre
  constraint coincident L4 L6.end
  constraint perpendicular L5 L6
  constraint tangent A0 L6
  measures "d107" diameter of A0
extrude "Extrude20" cut sketch "Sketch22" against normal blind 35 contours L2 A0 picked at (-9.0585, 15.7428) bodies 1
sketch "Sketch23" plane through (-43, 0, 0) normal (-1, 0, 0) x (0, -1, 0)
  line L0 (-40, 5) -> (40, 5)
  line L1 (40, 5) -> (40, 7)
  line L2 (40, 7) -> (32, 7)
  line L3 (32, 7) -> (32, 17)
  line L4 (32, 17) -> (-3, 17)
  line L5 (-3, 17) -> (-3, 7)
  line L6 (-3, 7) -> (-38, 7)
  line L7 (-38, 7) -> (-38, 160)
  line L8 (-38, 160) -> (-40, 160)
  line L9 (-40, 160) -> (-40, 5)
  line L10 (-3, 7) -> (32, 7)
  constraint coincident L5.end L6.start
  constraint coincident L2.end L3.start
extrude "Extrude21" cut sketch "Sketch23" against normal blind 10 contours L3 L4 L5 L10 bodies 1
sketch "Sketch24" plane through (43, 0, 0) normal (1, 0, 0) x (0, 1, 0)
  line L0 (-40, 5) -> (40, 5)
  line L1 (40, 5) -> (40, 160)
  line L2 (40, 160) -> (38, 160)
  line L3 (38, 160) -> (38, 7)
  line L4 (38, 7) -> (3, 7)
  line L5 (3, 7) -> (3, 17)
  line L6 (3, 17) -> (-32, 17)
  line L7 (-32, 17) -> (-32, 7)
  line L8 (-32, 7) -> (-40, 7)
  line L9 (-40, 7) -> (-40, 5)
  line L10 (-32, 7) -> (3, 7)
  constraint coincident L7.end L8.start
  constraint coincident L4.end L5.start
extrude "Extrude22" cut sketch "Sketch24" against normal blind 10 contours L5 L6 L7 L10 bodies 1
sketch "Sketch25" plane through (0, 0, 2) normal (0, 0, 1) x (-1, 0, 0)
  line L0 (-33, -3) -> (-33, 32)
  line L1 (-33, 32) -> (0, 32)
  line L2 (0, 32) -> (33, 32)
  line L3 (33, 32) -> (33, -3)
  line L4 (33, -3) -> (0, -3)
  line L5 (0, -3) -> (-33, -3)
  line L6 (31.9523, 36.4523) -> (31.9523, 41)
  line L7 (31.9523, 41) -> (-31.9523, 41)
  line L8 (-31.9523, 41) -> (-31.9523, 36.4523)
  arc A0 (-36.4523, 31.9523) -> (-31.9523, 36.4523) centre (-36.4523, 36.4523) ccw
  line L9 (-36.4523, 31.9523) -> (-41, 31.9523)
  line L10 (-41, 31.9523) -> (-41, -40)
  line L11 (-41, -40) -> (-40, -40)
  line L12 (-40, -40) -> (-40, -43)
  line L13 (-40, -43) -> (40, -43)
  line L14 (40, -43) -> (40, -40)
  line L15 (40, -40) -> (41, -40)
  line L16 (41, -40) -> (41, 31.9523)
  line L17 (41, 31.9523) -> (36.4523, 31.9523)
  arc A1 (31.9523, 36.4523) -> (36.4523, 31.9523) centre (36.4523, 36.4523) ccw
  line L18 (33, -3) -> (-33, -3)
  line L19 (-33, -3) -> (-33, -8)
  line L20 (-33, -8) -> (33, -8)
  line L21 (33, -8) -> (33, -3)
  dimension "d115" = 5
  constraint horizontal L18
  constraint vertical L19
  constraint horizontal L20
  constraint vertical L21
  constraint coincident L3.end L4.start
  measures "d115" distance of L3.end L20.end
fillet "Fillet6" radius 1.5 6 edges at (42, 45, 80) (45, 42, 80) (-42, 45, 80) (-45, 42, 80) (-42, 42, 80) (42, 42, 80) on bodies 1
sketch "Sketch31" plane through (0, 38, 0) normal (0, -1, 0) x (1, 0, 0)
  circle A0 centre (-38.265, 143.23) radius 1.65
  circle A1 centre (-38.165, 56.17) radius 1.65
  circle A2 centre (-37, 15) radius 2.15
  circle A3 centre (-37, 155) radius 2.15
  line L0 (-42, 150.5) -> (-37, 150.5)
  arc A4 (-37, 150.5) -> (-37, 159.5) centre (-37, 155) ccw
  line L1 (-37, 159.5) -> (-42, 159.5)
  line L2 (-42, 159.5) -> (-42, 160)
  line L3 (-42, 160) -> (-43, 160)
  line L4 (-43, 160) -> (-43, 7)
  line L5 (-43, 7) -> (-42, 7)
  line L6 (-42, 7) -> (-42, 10.5)
  line L7 (-42, 10.5) -> (-37, 10.5)
  arc A5 (-37, 10.5) -> (-37, 19.5) centre (-37, 15) ccw
  line L8 (-37, 19.5) -> (-42, 19.5)
  line L9 (-42, 19.5) -> (-42, 53.17)
  line L10 (-42, 53.17) -> (-38.165, 53.17)
  arc A6 (-38.165, 53.17) -> (-38.165, 59.17) centre (-38.165, 56.17) ccw
  line L11 (-38.165, 59.17) -> (-42, 59.17)
  line L12 (-42, 59.17) -> (-42, 140.23)
  line L13 (-42, 140.23) -> (-38.265, 140.23)
  arc A7 (-38.265, 140.23) -> (-38.265, 146.23) centre (-38.265, 143.23) ccw
  line L14 (-38.265, 146.23) -> (-42, 146.23)
  line L15 (-42, 146.23) -> (-42, 150.5)
  line L16 (-37, 15) -> (-43, 15) construction
  line L17 (-30, 20) -> (-44, 20)
  line L18 (-44, 20) -> (-44, 10)
  line L19 (-44, 10) -> (-30, 10)
  line L20 (-30, 10) -> (-30, 20)
  line L21 (-30, 20) -> (-44, 10) construction
  line L22 (-44, 20) -> (-30, 10) construction
  line L23 (0, 0) -> (0, 47) construction
  line L24 (30, 10) -> (30, 20)
  line L25 (30, 20) -> (44, 20)
  line L26 (44, 20) -> (44, 10)
  line L27 (44, 10) -> (30, 10)
  line L28 (-30, 160) -> (-44, 160)
  line L29 (-44, 160) -> (-44, 150)
  line L30 (-44, 150) -> (-30, 150)
  line L31 (-30, 150) -> (-30, 160)
  line L32 (30, 150) -> (30, 160)
  line L33 (30, 160) -> (44, 160)
  line L34 (44, 150) -> (30, 150)
  line L35 (44, 160) -> (44, 150)
  point P0 (-37, 15)
  dimension "d136" = 10
  dimension "d137" = 10
  constraint coincident P0 A2.centre
  constraint coincident L4 L16.end
  constraint perpendicular L4 L16
  constraint horizontal L17
  constraint perpendicular L17 L18
  constraint parallel L17 L19
  constraint parallel L18 L20
  constraint coincident L21 P0
  constraint coincident L22 P0
  constraint coincident L23.start origin
  constraint vertical L23
  constraint symmetric L17.start L23 L24.end
  constraint symmetric L17.end L23 L25.end
  constraint symmetric L18.end L23 L26.end
  constraint symmetric L19.end L23 L24.start
  constraint horizontal L28
  constraint perpendicular L28 L29
  constraint parallel L28 L30
  constraint parallel L29 L31
  measures "d136" distance of L17.end L18.end
  measures "d137" distance of L28.end L29.end
extrude "Extrude28" cut sketch "Sketch31" against normal blind 2 contours L0 A4 L1 L2 L3 L4 L15 L28 L30 | L0 A4 L1 L2 L15 L28 L30 L31 | L4 L28 L29 L30 | L4 L6 L7 A5 L8 L9 L17 L19 | L4 L17 L18 L19 | L6 L7 A5 L8 L9 L17 L19 L20 | L24 L25 L26 L27 | L32 L33 L34 L35 bodies 1
sketch "Sketch32" plane through (0, 0, 7) normal (0, 0, 1) x (-1, 0, 0)
  circle A0 centre (-36.4523, 36.4523) radius 2
  circle A1 centre (36.4523, 36.4523) radius 2
  line L0 (-43, 40) -> (-43, -38)
  line L1 (-43, -38) -> (-42, -38)
  line L2 (-42, -38) -> (-42, 31.9523)
  line L3 (-42, 31.9523) -> (-36.4523, 31.9523)
  arc A2 (-36.4523, 31.9523) -> (-31.9523, 36.4523) centre (-36.4523, 36.4523) ccw
  line L4 (-31.9523, 36.4523) -> (-31.9523, 42)
  line L5 (-31.9523, 42) -> (31.9523, 42)
  line L6 (31.9523, 42) -> (31.9523, 36.4523)
  arc A3 (31.9523, 36.4523) -> (36.4523, 31.9523) centre (36.4523, 36.4523) ccw
  line L7 (36.4523, 31.9523) -> (42, 31.9523)
  line L8 (42, 31.9523) -> (42, -38)
  line L9 (42, -38) -> (43, -38)
  line L10 (43, -38) -> (43, 40)
  line L11 (43, 40) -> (40, 40)
  line L12 (40, 40) -> (40, 43)
  line L13 (40, 43) -> (-40, 43)
  line L14 (-40, 43) -> (-40, 40)
  line L15 (-40, 40) -> (-43, 40)
  line L16 (0, 45) -> (0, 26) construction
  line L17 (29.4523, 29.4523) -> (43.4523, 29.4523)
  line L18 (43.4523, 29.4523) -> (43.4523, 43.4523)
  line L19 (43.4523, 43.4523) -> (29.4523, 43.4523)
  line L20 (29.4523, 43.4523) -> (29.4523, 29.4523)
  line L21 (29.4523, 29.4523) -> (43.4523, 43.4523) construction
  line L22 (43.4523, 29.4523) -> (29.4523, 43.4523) construction
  line L23 (37.3537, 29.4523) -> (29.4523, 35.2434)
  line L24 (-29.4523, 43.4523) -> (-29.4523, 29.4523)
  line L25 (-29.4523, 29.4523) -> (-43.4523, 29.4523)
  line L26 (-43.4523, 29.4523) -> (-43.4523, 43.4523)
  line L27 (-43.4523, 43.4523) -> (-29.4523, 43.4523)
  line L28 (-37.3537, 29.4523) -> (-29.4523, 35.2434)
  point P0 (36.4523, 36.4523)
  dimension "d140" = 14
  dimension "d141" = 14
  constraint vertical L16
  constraint horizontal L17
  constraint perpendicular L17 L18
  constraint parallel L17 L19
  constraint parallel L18 L20
  constraint coincident L21 P0
  constraint coincident L22 P0
  constraint coincident P0 A1.centre
  constraint coincident L17 L23.start
  constraint coincident L20 L23.end
  constraint symmetric L16 L17.start L24.end
  constraint symmetric L16 L17.end L25.end
  constraint symmetric L16 L18.end L26.end
  constraint symmetric L16 L19.end L24.start
  constraint symmetric L16 L23.start L28.start
  constraint symmetric L16 L23.end L28.end
  measures "d140" distance of L18.end L19.end
  measures "d141" distance of L17.end L18.end
extrude "Extrude29" cut sketch "Sketch32" against normal blind 2 contours L0 L2 L3 A2 L4 L5 L13 L14 L15 L24 L25 | L0 L13 L14 L15 L24 L25 L26 L27 | L2 L3 A2 L4 L5 L24 L25 L28 | L10 L11 L12 L13 L17 L18 L19 L20 | L5 L6 A3 L7 L8 L10 L11 L12 L13 L17 L20 | L5 L6 A3 L7 L8 L17 L20 L23 bodies 1
sketch "Sketch33" plane through (0, -32, 0) normal (0, -1, 0) x (1, 0, 0)
  line L0 (33, 2) -> (33, 17)
  line L1 (33, 17) -> (30.4959, 17)
  arc A0 (0, 2) -> (30.4959, 17) centre (0, 40.5) ccw
  line L2 (0, 2) -> (33, 2)
  line L3 (33, 2) -> (-33, 2) construction
  line L4 (-4, 2) -> (4, 2)
  line L5 (4, 2) -> (4, 45)
  line L6 (4, 45) -> (-4, 45)
  line L7 (-4, 45) -> (-4, 2)
  line L8 (0, 0) -> (0, 27) construction
  circle A1 centre (0, 40.5) radius 2.15
  line L9 (-4, 2) -> (4, 2)
  line L10 (4, 2) -> (4, 0)
  line L11 (4, 0) -> (-4, 0)
  line L12 (-4, 0) -> (-4, 2)
  dimension "d144" = 8
  dimension "d145" = 4
  dimension "d146" = 43
  dimension "d147" = 4.3
  constraint coincident L0.start L2.end
  constraint perpendicular L0 L3
  constraint horizontal L4
  constraint vertical L5
  constraint horizontal L6
  constraint vertical L7
  constraint coincident L3 L4.start
  constraint coincident L8.start origin
  constraint perpendicular L4 L8
  constraint concentric A0 A1
  constraint horizontal L9
  constraint vertical L10
  constraint horizontal L11
  constraint vertical L12
  measures "d144" distance of L5.end L6.end
  measures "d145" distance of L7 L8
  measures "d146" distance of L4.start L6.end
  measures "d147" diameter of A1
extrude "Extrude30" add sketch "Sketch33" along normal blind 5 separate body contours L2 L4 L9 L10 L11 L12 | A0 L2 L4 L5 L9 | A0 L4 L5 L6 L7 L9 makes body 2
combine "Combine1" operation add target body 2 tool bodies 1
chamfer "Chamfer3" distance 4 angle 45 2 edges at (-4, -34.5, 2) (4, -34.5, 2) on bodies 2
chamfer "Chamfer4" distance 4 angle 45 1 edges at (0, -37, 2) on bodies 2
equation "d71 = 1.7 mm + 1.5 mm"
equation "d72 = 1.7 mm + 1.5 mm"
equation "d74 = 1.2 mm + 1.5 mm"
equation "d75 = 1.8 mm + 1.5 mm"
equation "d77 = 1.2 mm + 1.5 mm"
equation "d78 = 1.55 mm + 1.5 mm"
equation "d80 = 1.3 mm + 1.5 mm"
equation "d81 = 1.2 mm + 1.5 mm"
